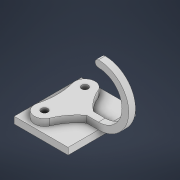
# Autodesk Inventor part: Pieza de practica 3
Saved by Autodesk Inventor 2022 (Build 260153000, 153)
## iProperties
Created: 2022-06-14
Part Number: Pieza de practica 3
Material: Genérico
Document SubType Name: Modeling
Designer: aleon
Density: 1 g/cm^3
Appearance: Valor por defecto
Author: aleon
Autodesk Inventor part; units mm, degrees
ref_plane "YZ Plane" through (0, 0, 0) normal (1, 0, 0) x (0, 1, 0)
ref_plane "XZ Plane" through (0, 0, 0) normal (0, 1, 0) x (-1, 0, 0)
ref_plane "XY Plane" through (0, 0, 0) normal (0, 0, 1) x (1, 0, 0)
sketch "Boceto1" plane through (0, 0, 0) normal (0, 1, 0) x (-1, 0, 0)
  line L0 (-8, -10) -> (8, -10)
  line L1 (8, -10) -> (8, 10)
  line L2 (8, 10) -> (-8, 10)
  line L3 (-8, 10) -> (-8, -10)
  point P0 (0, 0)
  dimension "d0" = 16
  dimension "d1" = 20
  constraints: 8 end point, 2 parallel, 1 horizontal, 1 perpendicular
  measures "d0" distance of L2.end L1.end
  measures "d1" distance of L1.end L0.end
extrude "Extrusión1" add sketch "Boceto1" along normal blind 2
sketch "Boceto2" plane through (0, 2, 0) normal (0, 1, 0) x (1, 0, 0)
  circle A0 centre (-3, -6) radius 1
  line L0 (-8, 10) -> (-8, -10) projected
  arc A1 (-5.8961, -5.2174) -> (-0.2307, -7.1538) centre (-3, -6) ccw
  arc A2 (4.5133, -1) -> (-0.2307, -7.1538) centre (13.6156, -12.9225) ccw
  line L1 (0, 0) -> (3.6811, 0) construction
  arc A3 (-0.2307, 7.1538) -> (-5.8961, 5.2174) centre (-3, 6) ccw
  arc A4 (-0.2307, 7.1538) -> (4.5133, 1) centre (13.6156, 12.9225) ccw
  arc A5 (-5.8961, -5.2174) -> (-5.8961, 5.2174) centre (-25.2036, 0) ccw
  circle A6 centre (-3, 6) radius 1
  line L2 (4.5133, -1) -> (8, -1)
  line L3 (8, -10) -> (8, 10) projected
  line L4 (4.5133, 1) -> (8, 1)
  dimension "d4" = 2
  dimension "d5" = 5
  dimension "d6" = 6
  dimension "d7" = 3
  dimension "d8" = 15
  dimension "d9" = 2
  dimension "d10" = 20
  dimension "d11" = 2
  constraints: 10 point on circle, 7 centre point, 6 end point, 5 symmetric about line, 2 coincident, 2 horizontal, 2 point on line, 2 tangent, 1 parallel, 2 other
  measures "d4" diameter of A0
  measures "d5" distance from line of A0.centre L0
  measures "d6" vertical distance of L1.start A0.centre
  measures "d7" radius of A1
  measures "d8" radius of A2
  measures "d9" distance of L4.start L2.start
  measures "d10" radius of A5
  measures "d11" diameter of A6
extrude "Extrusión2" add sketch "Boceto2" along normal blind 2
extrude "Extrusión3" cut sketch "Boceto2" against normal up to surface (2 mm away) contours A0 | A6
sketch "Boceto3" plane through (0, 0, 0) normal (0, 0, 1) x (1, 0, 0)
  line L0 (8, 0) -> (8, 2) construction
  line L1 (8, 0) -> (8, 22) construction
  arc A0 (8, 2) -> (8, 20) centre (8, 11) ccw
  line L2 (4.5133, 4) -> (8, 4) projected
  arc A1 (8, 4) -> (8, 18) centre (8, 11) ccw
  arc A2 (8, 20) -> (8, 18) centre (8, 19) ccw
  point P0 (0, 0)
  dimension "d16" = 9
  dimension "d17" = 7
  dimension "d18" = 2
  dimension "d19" = 1
  constraints: 6 point on circle, 3 centre point, 2 end point, 2 point on line, 1 midpoint, 1 vertical
  measures "d16" radius of A0
  measures "d17" radius of A1
  measures "d18" distance of A0.end A1.end
  measures "d19" radius of A2
extrude "Extrusión4" add sketch "Boceto3" along normal mid plane 2 fills toward (15.05, 11) open curves A1 A2 A0
